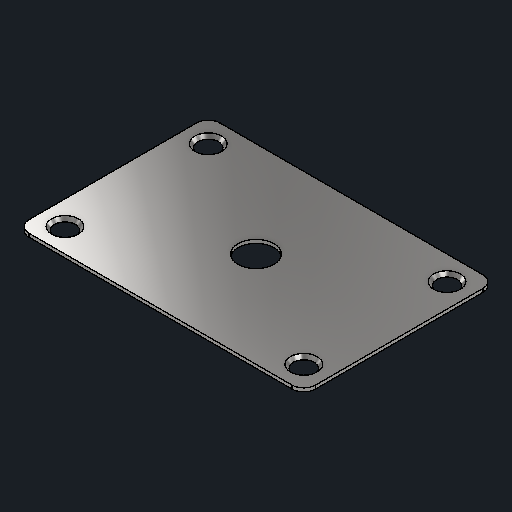
# Autodesk Inventor part: Jack Plate
Saved by Autodesk Inventor 2026.2 (Build 302298000, 298)
## iProperties
Created: 2026-06-24
Part Number: Jack Plate
Material: Steel, Carbon
Document SubType Name: Sheet Metal
Designer: JoshuaEah
Density: 7.85 g/cm^3
Sheet Metal Rule: 20 Gauge (0.0359") Carbon Steel Sheet A1008
Appearance: Semi-Polished
Author: JoshuaEah
Autodesk Inventor part; units mm, degrees
ref_plane "YZ Plane" through (0, 0, 0) normal (1, 0, 0) x (0, 1, 0)
ref_plane "XZ Plane" through (0, 0, 0) normal (0, 1, 0) x (-1, 0, 0)
ref_plane "XY Plane" through (0, 0, 0) normal (0, 0, 1) x (1, 0, 0)
sketch "Profile" plane through (0, 0, 0) normal (0, 1, 0) x (-1, 0, 0)
  line L0 (0, 0) -> (-76.2, 0)
  line L1 (-76.2, 0) -> (-76.2, -50.8)
  line L2 (-76.2, -50.8) -> (0, -50.8)
  line L3 (0, -50.8) -> (0, 0)
  line L4 (0, -25.4) -> (-76.2, -25.4)
  line L5 (-38.1, -50.8) -> (-38.1, 0)
  line L6 (-6.35, -44.45) -> (-69.85, -44.45) construction
  line L7 (-69.85, -44.45) -> (-69.85, -6.35) construction
  line L8 (-69.85, -6.35) -> (-6.35, -6.35) construction
  line L9 (-6.35, -6.35) -> (-6.35, -44.45) construction
  line L10 (-6.35, -44.45) -> (-69.85, -6.35) construction
  line L11 (-69.85, -44.45) -> (-6.35, -6.35) construction
  circle A0 centre (-38.1, -25.4) radius 4.5
  dimension "d0" = 76.2
  dimension "d1" = 50.8
  dimension "d2" = 63.5
  dimension "d3" = 38.1
  dimension "d13" = 9
  constraints: 24 end point, 7 midpoint, 5 coincident, 4 parallel, 2 horizontal, 2 perpendicular, 2 point on line, 1 centre point
  measures "d0" distance of L2.end L1.end
  measures "d1" distance of L1.end L0.end
  measures "d2" distance of L7.end L8.end
  measures "d3" distance of L6.end L7.end
  measures "d13" diameter of A0
extrude "Plate1" add sketch "Profile" against normal blind 0.9119
hole "#6 Mounting Hole" at (6.35, 0, -44.45) direction (0, -1, 0) diameter 3.81 end through all start extended yes countersink diameter 7.0866 countersink angle 82 clearance for "Flat Head Machine Screw (82)" size "#6" standard "Ansi Unified Screw Threads"
pattern_sketch "Jack Plate Mounting Holes" of "#6 Mounting Hole" from (6.35, 0, -44.45) copies at (69.85, 0, -44.45) at (69.85, 0, -6.35) at (6.35, 0, -6.35)
hole "Input Jack Hole" at (38.1, 0, -25.4) direction (0, -1, 0) diameter 9.525 end through all start extended yes
fillet "Corner Round1" radius 3.175 4 edges at (0, -0.4559, -50.8) (76.2, -0.4559, -50.8) (76.2, -0.4559, 0) (0, -0.4559, 0)
equation "\"d11\" = Thickness"
equation "\"d5\" = Thickness"
equation "\"BendRadius\" = Thickness"
equation "\"BendReliefWidth\" = Thickness"
equation "\"BendReliefDepth\" = 0.5 * Thickness"
equation "\"CornerReliefSize\" = 4 * Thickness"
equation "\"MinimumRemnant\" = 2 * Thickness"
equation "\"TransitionRadius\" = BendRadius"
equation "\"JacobiRadiusSize\" = BendRadius"
equation "\"GapSize\" = Thickness"
equation "\"Thickness\" = 0.91186"
body "Solid1"
